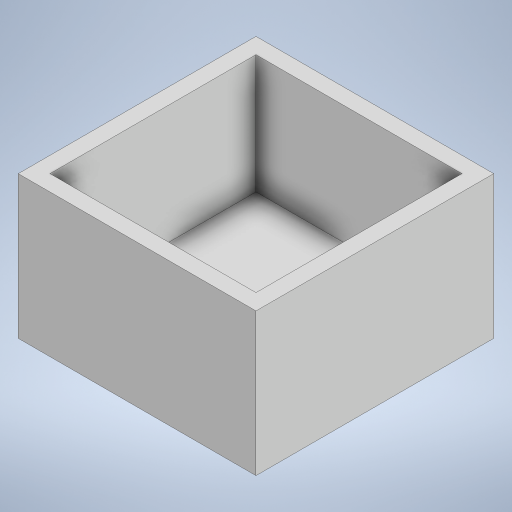
# Autodesk Inventor part: Boks
Saved by Autodesk Inventor 2023 (Build 270158000, 158)
## iProperties
Created: 2023-04-11
Part Number: Boks
Material: Generic
Document SubType Name: Modeling
Designer: Anders
Density: 1 g/cm^3
Appearance: Default
Author: Anders
## iProperties of the stored document Boks_3DPrint.ipt
Created: 2023-04-11
Part Number: Boks_3DPrint
Material: Generic
Document SubType Name: Modeling
Designer: Anders
Density: 1 g/cm^3
Appearance: Default
Author: Anders
Autodesk Inventor part; units mm, degrees
ref_plane "YZ Plane" through (0, 0, 0) normal (1, 0, 0) x (0, 1, 0)
ref_plane "XZ Plane" through (0, 0, 0) normal (0, 1, 0) x (-1, 0, 0)
ref_plane "XY Plane" through (0, 0, 0) normal (0, 0, 1) x (1, 0, 0)
sketch "Sketch1" plane through (0, 0, 0) normal (0, 1, 0) x (-1, 0, 0)
  line L0 (0, 0) -> (30, 0)
  line L1 (30, 0) -> (30, -30)
  line L2 (30, -30) -> (0, -30)
  line L3 (0, -30) -> (0, 0)
  line L4 (28, -2) -> (2, -2)
  line L5 (2, -2) -> (2, -28)
  line L6 (2, -28) -> (28, -28)
  line L7 (28, -28) -> (28, -2)
  point P0 (0, -15)
  point P1 (2, -15)
  dimension "d0" = 30
  dimension "d1" = 30
  dimension "d2" = 2
  dimension "d3" = 2
  dimension "d4" = 2
  dimension "d5" = 2
  constraints: 16 end point, 4 parallel, 2 horizontal, 2 midpoint, 2 perpendicular
  measures "d0" distance of L1.end L2.end
  measures "d1" distance of L0.end L1.end
  measures "d2" distance between parallel lines of L1 L7
  measures "d3" distance between parallel lines of L0 L4
  measures "d4" distance of point (0, -15) point (2, -15)
  measures "d5" distance between parallel lines of L2 L6
extrude "Extrusion1" add sketch "Sketch1" along normal blind 15
sketch "Sketch2" plane through (0, 0, 0) normal (0, -1, 0) x (1, 0, 0)
  line L0 (-30, 0) -> (0, 0) projected
  line L1 (0, -30) -> (-30, -30) projected
  line L2 (-30, 0) -> (0, 0)
  line L3 (0, 0) -> (0, -30)
  line L4 (0, -30) -> (-30, -30)
  line L5 (-30, -30) -> (-30, 0)
  constraints: 8 end point, 2 parallel, 1 horizontal, 1 perpendicular
extrude "Extrusion2" add sketch "Sketch2" along normal blind 3
body "Solid1"
